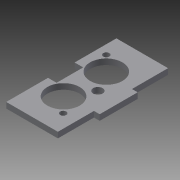
# Autodesk Inventor part: srf
Saved by Autodesk Inventor 2014 (Build 180170000, 170)
## iProperties
Created: 2014-12-05
Part Number: srf
Material: Generic
Document SubType Name: Modeling
Designer: Yosua
Density: 1 g/cm^3
Appearance: Default
Author: Yosua
Autodesk Inventor part; units mm, degrees
ref_plane "YZ Plane" through (0, 0, 0) normal (1, 0, 0) x (0, 1, 0)
ref_plane "XZ Plane" through (0, 0, 0) normal (0, 1, 0) x (-1, 0, 0)
ref_plane "XY Plane" through (0, 0, 0) normal (0, 0, 1) x (1, 0, 0)
sketch "Sketch1" plane through (0, 0, 0) normal (0, 0, 1) x (1, 0, 0)
  circle A0 centre (-14.6869, 39.4735) radius 8.5
  circle A1 centre (-22.3409, 47.1275) radius 1.6
  circle A2 centre (-7.0512, 9.17) radius 1.6
  circle A3 centre (-8.1473, 28.508) radius 2.5
  circle A4 centre (-14.6869, 16.9735) radius 8.5
  line L0 (0, 28.315) -> (0, -0.685)
  line L1 (0, -0.685) -> (-27.2, -0.685)
  line L2 (-27.2, -0.685) -> (0, -0.685)
  line L3 (0, -0.685) -> (0, 57.315)
  line L4 (0, 57.315) -> (-27.2, 57.315)
  line L5 (-27.2, 57.315) -> (-27.2, -0.685)
  line L6 (0, 28.315) -> (0, 38.315)
  line L7 (0, 38.315) -> (3, 38.315)
  line L8 (3, 38.315) -> (3, 18.315)
  line L9 (3, 18.315) -> (0, 18.315)
  line L10 (-14.6869, 39.4735) -> (-14.6869, 28.315)
  line L11 (-14.6869, 28.315) -> (-22.6869, 28.315)
  line L12 (-22.6869, 28.315) -> (-22.6869, 21.315)
  line L13 (-22.6869, 21.315) -> (-22.6869, 35.315)
  line L14 (-22.6869, 35.315) -> (-27.2, 35.315)
  line L15 (-22.6869, 21.315) -> (-27.2, 21.315)
  point P0 (0, 0)
  point P1 (-5.6598, 20.3223)
  dimension "d1" = 29
  dimension "d2" = 58
  dimension "d3" = 10
  dimension "d4" = 3
  dimension "d5" = 20
  dimension "d10" = 8
  dimension "d11" = 7
  dimension "d12" = 14
  constraints: 32 end point, 8 perpendicular, 5 centre point, 4 parallel, 4 point on line, 1 collinear, 1 horizontal
  measures "d1" distance of L0.start L0.end
  measures "d2" distance of L3.end L2.end
  measures "d3" distance of L0.start L6.end
  measures "d4" distance of L6.end L7.end
  measures "d5" distance of L7.end L8.end
  measures "d10" distance of L10.end L11.end
  measures "d11" distance of L11.end L12.end
  measures "d12" distance of L12.end L13.end
extrude "Extrusion2" add sketch "Sketch1" along normal blind 3 contours L3 L7 L8 L9 L0 | L0 L1 L5 L15 L12 L13 L14 L4 L3
body "Solid2"
